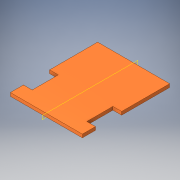
# Autodesk Inventor part: BasePlate
Saved by Autodesk Inventor 2016 SP1 (Build 200210100, 210)
## iProperties
Created: 2015-12-30
Part Number: BasePlate
Material: Wood (Walnut)
Document SubType Name: Modeling
Designer: steele
Density: 0.55 g/cm^3
Appearance: Walnut - Natural Polished
Mass: 3217.6 g
Surface Area: 6616.12 cm^2
Volume: 5850.18 cm^3
Author: steele
Autodesk Inventor part; units mm, degrees
ref_plane "YZ Plane" through (0, 0, 0) normal (1, 0, 0) x (0, 1, 0)
ref_plane "XZ Plane" through (0, 0, 0) normal (0, 1, 0) x (-1, 0, 0)
ref_plane "XY Plane" through (0, 0, 0) normal (0, 0, 1) x (1, 0, 0)
sketch "Sketch1" plane through (0, 0, 0) normal (0, 1, 0) x (-1, 0, 0)
  line L0 (-209.55, 254) -> (-209.55, -254)
  line L1 (-209.55, -254) -> (209.55, -254)
  line L2 (209.55, -254) -> (209.55, 254)
  line L3 (209.55, 254) -> (-209.55, 254)
  line L4 (-209.55, 254) -> (209.55, -254) construction
  line L5 (-209.55, -254) -> (209.55, 254) construction
  point P0 (0, 0)
  dimension "baseLength" = 508
  dimension "baseWidth" = 419.1
  constraints: 12 end point, 2 midpoint, 2 parallel, 1 perpendicular, 1 vertical
  measures "baseLength" distance of L0.start L0.end
  measures "baseWidth" distance of L2.end L0.start
extrude "Extrusion1" add sketch "Sketch1" along normal blind 19.05
sketch "Sketch2" plane through (0, 0, 0) normal (0, -1, 0) x (1, 0, 0)
  line L0 (209.55, 254) -> (209.55, -254) projected
  line L1 (209.55, 177.8) -> (158.75, 177.8)
  line L2 (158.75, 177.8) -> (158.75, 25.4)
  line L3 (158.75, 25.4) -> (209.55, 25.4)
  line L4 (209.55, 25.4) -> (209.55, 177.8)
  line L5 (-209.55, 254) -> (209.55, 254) projected
  point P0 (0, 0)
  dimension "backToEndOfGearBox" = 76.2
  dimension "backToFrontOfGearBox" = 228.6
  dimension "wdithForGearBox" = 50.8
  constraints: 8 end point, 2 perpendicular, 2 point on line, 1 collinear, 1 horizontal
  measures "backToEndOfGearBox" distance between parallel lines of L1 L5
  measures "backToFrontOfGearBox" distance between parallel lines of L3 L5
  measures "wdithForGearBox" distance between parallel lines of L2 L0
extrude "Extrusion2" cut sketch "Sketch2" against normal through all
mirror "Mirror1" about plane through (0, 0, 0) normal (1, 0, 0) of "Extrusion2"
body "Solid1"
